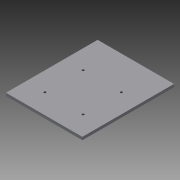
# Autodesk Inventor part: backPlate
Saved by Autodesk Inventor 2013 (Build 170138000, 138)
## iProperties
Created: 2012-12-09
Part Number: backPlate
Material: Generic
Document SubType Name: Modeling
Designer: Istvan
Density: 1 g/cm^3
Author: Istvan
Autodesk Inventor part; units mm, degrees
ref_plane "YZ Plane" through (0, 0, 0) normal (1, 0, 0) x (0, 1, 0)
ref_plane "XZ Plane" through (0, 0, 0) normal (0, 1, 0) x (-1, 0, 0)
ref_plane "XY Plane" through (0, 0, 0) normal (0, 0, 1) x (1, 0, 0)
sketch "Sketch1" plane through (0, 0, 0) normal (0, 1, 0) x (-1, 0, 0)
  line L0 (0, 0) -> (127, 0)
  line L1 (127, 0) -> (127, 152.4)
  line L2 (127, 152.4) -> (0, 152.4)
  line L3 (0, 152.4) -> (0, 0)
  dimension "d0" = 127
  dimension "d1" = 152.4
  constraints: 8 end point, 2 parallel, 1 horizontal, 1 perpendicular
  measures "d0" distance of L2.end L1.end
  measures "d1" distance of L1.end L0.end
extrude "Extrusion1" add sketch "Sketch1" against normal blind 4.7625
sketch "Sketch2" plane through (0, 0, 0) normal (0, 1, 0) x (1, 0, 0)
  line L0 (0, 0) -> (-127, 0) projected
  line L1 (-127, 0) -> (-127, -152.4) projected
  line L2 (0, -152.4) -> (0, 0) projected
  point P0 (-95.25, -55.88)
  point P1 (-31.75, -55.88)
  point P2 (-95.25, -119.38)
  point P3 (-31.75, -119.38)
  dimension "d4" = 63.5
  dimension "d6" = 31.75
  dimension "d8" = 31.75
  dimension "d9" = 63.5
  dimension "d10" = 55.88
  constraints: 2 horizontal alignment, 2 vertical alignment
  measures "d4" distance of point (-31.75, -55.88) point (-95.25, -55.88)
  measures "d6" distance from line of L1 point (-95.25, -55.88)
  measures "d8" distance from line of L2 point (-31.75, -55.88)
  measures "d9" distance of point (-95.25, -119.38) point (-95.25, -55.88)
  measures "d10" distance from line of L0 point (-95.25, -55.88)
hole "Hole1" at (-95.25, 0, 55.88) at (-31.75, 0, 55.88) at (-95.25, 0, 119.38) at (-31.75, 0, 119.38) direction (0, -1, 0) diameter 3.683 end through all thread size "10-24 UNC" class "2B" standard "ANSI Unified Screw Threads"
equation "\"d6\" = d8"
body "Solid1"
